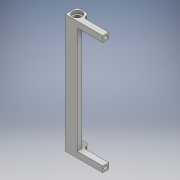
# Autodesk Inventor part: rearAxelHolder 6-5
Saved by Autodesk Inventor 2018 (Build 220112000, 112)
## iProperties
Created: 2019-06-05
Part Number: rearAxelHolder 6-5
Material: Generic
Document SubType Name: Modeling
Designer: Aditya Kendre
Density: 1 g/cm^3
Appearance: Default
Author: Aditya Kendre
Autodesk Inventor part; units mm, degrees
ref_plane "YZ Plane" through (0, 0, 0) normal (1, 0, 0) x (0, 1, 0)
ref_plane "XZ Plane" through (0, 0, 0) normal (0, 1, 0) x (-1, 0, 0)
ref_plane "XY Plane" through (0, 0, 0) normal (0, 0, 1) x (1, 0, 0)
sketch "Sketch1" plane through (0, 0, 0) normal (1, 0, 0) x (0, 1, 0)
  line L0 (0, 0) -> (10, 0)
  line L1 (10, 0) -> (10, -200)
  line L2 (10, -200) -> (0, -200)
  line L3 (0, -200) -> (0, 0)
  dimension "d0" = 10
  dimension "d1" = 200
  constraints: 8 end point, 2 parallel, 1 horizontal, 1 perpendicular
  measures "d0" distance of L1.end L2.end
  measures "d1" distance of L0.end L1.end
extrude "Extrusion1" add sketch "Sketch1" along normal blind 3
sketch "Sketch2" plane through (3, 0, 0) normal (1, 0, 0) x (0, 0, -1)
  line L0 (0, 10) -> (0, 0) projected
  line L1 (0, 0) -> (200, 0) projected
  line L2 (0, 10) -> (10, 10)
  line L3 (10, 10) -> (10, 0)
  line L4 (10, 0) -> (0, 0)
  line L5 (0, 0) -> (0, 10)
  line L6 (200, 0) -> (200, 10) projected
  line L7 (200, 10) -> (190, 10)
  line L8 (190, 10) -> (190, 0)
  line L9 (190, 0) -> (200, 0)
  line L10 (200, 0) -> (200, 10)
  dimension "d4" = 10
  dimension "d5" = 10
  constraints: 16 end point, 4 parallel, 2 horizontal, 2 perpendicular, 2 point on line
  measures "d4" distance of L3.end L4.end
  measures "d5" distance of L9.end L8.end
extrude "Extrusion2" add sketch "Sketch2" along normal blind 60
sketch "Sketch3" plane through (63, 0, 0) normal (1, 0, 0) x (0, 0, -1)
  line L0 (0, 10) -> (200, 10) construction
  line L1 (10, 0) -> (190, 0) construction
  line L2 (0, 10) -> (10, 0) construction
  line L3 (5, 5) -> (0, 5) construction
  line L4 (0, 0) -> (0, 10) construction
  circle A0 centre (5, 5) radius 3.175
  line L5 (200, 10) -> (190, 10) construction
  line L6 (200, 0) -> (200, 10) construction
  line L7 (190, 10) -> (200, 0) construction
  circle A1 centre (195, 5) radius 3.175
  dimension "d8" = 6.35
  dimension "d9" = 6.35
  constraints: 6 end point, 3 midpoint, 2 centre point, 1 coincident
  measures "d8" diameter of A0
  measures "d9" diameter of A1
extrude "Extrusion3" cut sketch "Sketch3" against normal blind 30
sketch "Sketch4" plane through (0, 0, -200) normal (0, 0, -1) x (-1, 0, 0)
  line L0 (0, 0) -> (-63, 0) construction
  line L1 (0, 0) -> (-20, 0) construction
  line L2 (-20, 0) -> (-20, 20) construction
  line L3 (-20, 20) -> (0, 20) construction
  line L4 (0, 20) -> (0, 0) construction
  line L5 (-3, 10) -> (-63, 10) construction
  circle A0 centre (-10, 10) radius 8 construction
  line L6 (0, 10) -> (-63, 10) projected
  arc A1 (-2, 10) -> (-18, 10) centre (-10, 10) ccw
  line L7 (-20, 10) -> (-18, 10)
  line L8 (-2, 10) -> (0, 10)
  line L9 (0, 20) -> (-20, 20)
  line L10 (-20, 10) -> (-20, 20)
  line L11 (0, 20) -> (0, 10)
  dimension "d12" = 20
  dimension "d13" = 20
  dimension "d14" = 16
  constraints: 18 end point, 5 collinear, 4 point on circle, 4 point on line, 2 centre point, 2 parallel, 1 concentric, 1 horizontal, 1 midpoint, 1 perpendicular
  measures "d12" distance of L2.end L3.end
  measures "d13" distance of L1.end L2.end
  measures "d14" diameter of A0
extrude "Extrusion4" add sketch "Sketch4" against normal blind 10 contours L6 A1 L10 L9 L11
fillet "Fillet1" radius 5 2 edges at (0, 20, -195) (20, 20, -195)
fillet "Fillet2" radius 5 1 edges at (20, 10, -195)
sketch "Sketch5" plane through (63, 0, -200) normal (0, 0, -1) x (-1, 0, 0)
  arc A0 (61, 10) -> (45, 10) centre (53, 10) ccw projected
  circle A1 centre (53, 10) radius 8
  point P0 (63, 0)
  constraints: 1 centre point, 1 coincident
extrude "Extrusion5" cut sketch "Sketch5" against normal blind 200
sketch "Sketch6" plane through (3, 0, -190) normal (0, 0, 1) x (1, 0, 0)
  arc A0 (0, 6.127) -> (-1, 10) centre (7, 10) ccw projected
  circle A1 centre (7, 10) radius 8
  circle A2 centre (7, 10) radius 5
  point P0 (-3, 0)
  dimension "d21" = 10
  constraints: 2 centre point, 2 coincident
  measures "d21" diameter of A2
extrude "Extrusion6" add sketch "Sketch6" against normal blind 5
sketch "Sketch7" plane through (0, 0, 0) normal (0, 0, 1) x (1, 0, 0)
  line L0 (0, 0) -> (63, 0) construction
  line L1 (0, 0) -> (20, 0) construction
  line L2 (20, 0) -> (20, 20) construction
  line L3 (20, 20) -> (0, 20) construction
  line L4 (0, 20) -> (0, 0) construction
  circle A0 centre (10, 10) radius 8 construction
  line L5 (2, 10) -> (0, 10) projected
  line L6 (2, 10) -> (0, 10)
  line L7 (0, 10) -> (0, 20)
  line L8 (20, 20) -> (0, 20)
  line L9 (20, 20) -> (20, 10)
  line L10 (18, 10) -> (63, 10) projected
  line L11 (18, 10) -> (20, 10)
  arc A1 (18, 10) -> (2, 10) centre (10, 10) ccw
  dimension "d24" = 20
  dimension "d25" = 20
  dimension "d26" = 16
  constraints: 18 end point, 4 collinear, 2 centre point, 2 parallel, 2 point on circle, 1 horizontal, 1 midpoint, 1 perpendicular, 1 point on line
  measures "d24" distance of L3.end L2.end
  measures "d25" distance of L2.end L1.end
  measures "d26" diameter of A0
extrude "Extrusion7" add sketch "Sketch7" against normal blind 10
fillet "Fillet3" radius 5 3 edges at (0, 20, -5) (20, 20, -5) (20, 10, -5)
sketch "Sketch8" plane through (63, 0, -10) normal (0, 0, -1) x (-1, 0, 0)
  circle A0 centre (53, 10) radius 5 projected
  circle A1 centre (53, 10) radius 5
  circle A2 centre (53, 10) radius 8
  point P0 (63, 0)
  constraints: 2 centre point, 2 coincident
extrude "Extrusion8" add sketch "Sketch8" against normal blind 5
sketch "Sketch9" plane through (63, 0, -10) normal (0, 0, -1) x (-1, 0, 0)
  line L0 (63, 0) -> (43, 0)
  line L1 (43, 0) -> (43, 2)
  line L2 (43, 2) -> (63, 2)
  line L3 (63, 2) -> (63, 0)
  dimension "d32" = 20
  dimension "d33" = 2
  constraints: 8 end point, 2 parallel, 1 horizontal, 1 perpendicular
  measures "d32" distance of L1.end L2.end
  measures "d33" distance of L0.end L1.end
extrude "Extrusion9" add sketch "Sketch9" along normal blind 190
sketch "Sketch10" plane through (3, 2, -10) normal (0, 1, 0) x (1, 0, 0)
  line L0 (17, 180) -> (14, 180)
  line L1 (14, 180) -> (14, 0)
  line L2 (14, 0) -> (17, 0)
  line L3 (17, 0) -> (17, 180)
  point P0 (-3, -10)
  dimension "d36" = 3
  constraints: 8 end point, 2 parallel, 1 horizontal, 1 perpendicular
  measures "d36" distance of L2.end L1.end
sketch "Sketch11" plane through (0, 10, -10) normal (0, 1, 0) x (1, 0, 0)
  line L0 (3, 180) -> (3, 0) projected
  line L1 (0, 180.0445) -> (3, 180.0445)
  line L2 (3, 180.0445) -> (3, 0)
  line L3 (3, 0) -> (0, 0)
  line L4 (0, 0) -> (0, 180.0445)
  point P0 (0, -10)
  constraints: 8 end point, 2 parallel, 1 horizontal, 1 perpendicular
extrude "Extrusion10" add sketch "Sketch11" against normal blind 10
extrude "Extrusion11" add sketch "Sketch10" along normal blind 6
body "Solid1"
